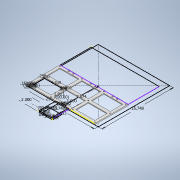
# Autodesk Inventor part: WellPlateFrame - 3L - Part2
Saved by Autodesk Inventor 2020 (Build 240168000, 168)
## iProperties
Created: 2023-02-18
Part Number: WellPlateFrame - 3L - Part2
Material: Generic
Document SubType Name: Modeling
Designer: Beaucage
Density: 1 g/cm^3
Appearance: Default
Author: Beaucage
Autodesk Inventor part; units mm, degrees
ref_plane "YZ Plane" through (0, 0, 0) normal (1, 0, 0) x (0, 1, 0)
ref_plane "XZ Plane" through (0, 0, 0) normal (0, 1, 0) x (-1, 0, 0)
ref_plane "XY Plane" through (0, 0, 0) normal (0, 0, 1) x (1, 0, 0)
sketch "Sketch1" plane through (0, 0, 0) normal (0, 1, 0) x (-1, 0, 0)
  line L0 (0, 0) -> (76.2, 0)
  line L1 (76.2, 0) -> (76.2, -50.8)
  line L2 (76.2, -50.8) -> (0, -50.8)
  line L3 (0, -50.8) -> (0, 0)
  line L4 (38.1, 0) -> (38.1, -6.35)
  line L5 (38.1, -6.35) -> (12.7, -6.35)
  line L6 (38.1, -6.35) -> (63.5, -6.35)
  line L7 (38.1, -6.35) -> (63.5, -6.35) construction
  line L8 (63.5, -6.35) -> (63.5, -19.05)
  line L9 (12.7, -6.35) -> (12.7, -19.05)
  line L10 (63.5, -19.05) -> (63.5, -25.4)
  line L11 (12.7, -19.05) -> (12.7, -25.4)
  line L12 (63.5, -19.05) -> (63.5, -94.05)
  line L13 (63.5, -19.05) -> (138.5, -19.05) construction
  line L14 (12.7, -19.05) -> (12.7, -94.05)
  line L15 (63.5, -94.05) -> (38.1, -94.05)
  line L16 (38.1, -94.05) -> (38.1, -294.05)
  line L17 (38.1, -94.05) -> (238.1, -94.05) construction
  line L18 (238.1, -494.05) -> (-161.9, -494.05)
  line L19 (-161.9, -494.05) -> (-161.9, -94.05)
  line L20 (-161.9, -94.05) -> (238.1, -94.05)
  line L21 (238.1, -94.05) -> (238.1, -494.05)
  line L22 (238.1, -494.05) -> (-161.9, -94.05) construction
  line L23 (-161.9, -494.05) -> (238.1, -94.05) construction
  point P0 (63.5, -50.8)
  point P1 (12.7, -50.8)
  dimension "d0" = 76.2
  dimension "d1" = 50.8
  dimension "d2" = 6.35
  dimension "d3" = 25.4
  dimension "d4" = 25.4
  dimension "d5" = 0
  dimension "d6" = 12.7
  dimension "d7" = 12.7
  dimension "d8" = 6.35
  dimension "d9" = 6.35
  dimension "d10" = 75
  dimension "d11" = 90
  dimension "d12" = 75
  dimension "d13" = 25.4
  dimension "d14" = 200
  dimension "d15" = 90
  dimension "d16" = 400
  dimension "d17" = 400
  constraints: 48 end point, 7 horizontal, 6 vertical, 4 parallel, 4 perpendicular, 3 equal length, 3 midpoint, 1 point on line
  measures "d0" distance of L1.end L2.end
  measures "d1" distance of L0.end L1.end
  measures "d2" distance of L4.start L4.end
  measures "d3" distance of L4.end L5.end
  measures "d4" distance of L4.end L6.end
  measures "d5" distance between parallel lines of L6 L7
  measures "d6" distance of L6.end L8.end
  measures "d7" distance of L5.end L9.end
  measures "d8" distance of L8.end L10.end
  measures "d9" distance of L9.end L11.end
  measures "d10" distance of L8.end L12.end
  measures "d11" angle of L12 L13
  measures "d12" distance of L9.end L14.end
  measures "d13" distance of L12.end L15.end
  measures "d14" distance of L15.end L16.end
  measures "d15" angle of L16 L17
  measures "d16" distance of L19.end L20.end
  measures "d17" distance of L18.end L19.end
extrude "Extrusion1" add sketch "Sketch1" along normal blind 6.35
hole "Hole1" at (-12.7, 0, -6.35) at (-12.7, 0, -19.05) at (-63.5, 0, -6.35) at (-63.5, 0, -19.05) direction (0, 1, 0) diameter 6.604 end through all
sketch "Sketch2" plane through (0, 0, 0) normal (0, -1, 0) x (1, 0, 0)
  line L0 (-238.1, -94.05) -> (-63.5, -94.05) projected
  line L1 (-238.1, -94.05) -> (-238.1, -100.4)
  line L2 (-238.1, -94.05) -> (-231.75, -94.05) construction
  line L3 (-238.1, -100.4) -> (-231.75, -100.4)
  line L4 (-231.75, -100.4) -> (-225.4, -100.4)
  line L5 (-225.4, -100.4) -> (-225.4, -106.75)
  line L6 (-225.4, -106.75) -> (-115.2, -106.75)
  line L7 (-115.2, -106.75) -> (-115.2, -180.75)
  line L8 (-115.2, -180.75) -> (-225.4, -180.75)
  line L9 (-225.4, -180.75) -> (-225.4, -106.75)
  line L10 (-115.2, -106.75) -> (-115.2, -100.4)
  line L11 (-115.2, -100.4) -> (-108.85, -100.4)
  line L12 (-225.4, -180.75) -> (-231.75, -180.75)
  line L13 (-231.75, -180.75) -> (-231.75, -187.1)
  line L14 (-115.2, -180.75) -> (-115.2, -187.1)
  line L15 (-115.2, -187.1) -> (-108.85, -187.1)
  line L16 (-225.4, -106.75) -> (-225.4, -114.75)
  line L17 (-225.4, -106.75) -> (-217.4, -106.75) construction
  line L18 (-225.4, -106.75) -> (-223.4, -106.75)
  line L19 (-223.4, -106.75) -> (-223.4, -108.75)
  line L20 (-223.4, -108.75) -> (-225.4, -108.75)
  line L21 (-225.4, -108.75) -> (-225.4, -106.75)
  line L22 (-115.2, -180.75) -> (-117.2, -180.75)
  line L23 (-117.2, -180.75) -> (-117.2, -178.75)
  line L24 (-117.2, -178.75) -> (-115.2, -178.75)
  line L25 (-115.2, -178.75) -> (-115.2, -180.75)
  line L26 (-223.4, -108.75) -> (-117.2, -108.75)
  line L27 (-117.2, -108.75) -> (-117.2, -178.75)
  line L28 (-117.2, -178.75) -> (-223.4, -178.75)
  line L29 (-223.4, -178.75) -> (-223.4, -108.75)
  point P0 (0, 0)
  dimension "d27" = 6.35
  dimension "d28" = 90
  dimension "d29" = 6.35
  dimension "d30" = 6.35
  dimension "d31" = 6.35
  dimension "d32" = 110.2
  dimension "d33" = 74
  dimension "d34" = 6.35
  dimension "d35" = 6.35
  dimension "d36" = 6.35
  dimension "d37" = 6.35
  dimension "d38" = 6.35
  dimension "d39" = 8
  dimension "d40" = 90
  dimension "d41" = 2
  dimension "d42" = 2
  dimension "d43" = 2
  dimension "d44" = 2
  constraints: 58 end point, 11 perpendicular, 8 horizontal, 8 parallel, 4 vertical
  measures "d27" distance of L0.start L1.end
  measures "d28" angle of L1 L2
  measures "d29" distance of L1.end L3.end
  measures "d30" distance of L3.end L4.end
  measures "d31" distance of L4.end L5.end
  measures "d32" distance of L7.end L8.end
  measures "d33" distance of L6.end L7.end
  measures "d34" distance of L10.end L11.end
  measures "d35" distance of L8.end L12.end
  measures "d36" distance of L12.end L13.end
  measures "d37" distance of L7.end L14.end
  measures "d38" distance of L14.end L15.end
  measures "d39" distance of L5.end L16.end
  measures "d40" angle of L16 L17
  measures "d41" distance of L19.end L20.end
  measures "d42" distance of L18.end L19.end
  measures "d43" distance of L23.end L24.end
  measures "d44" distance of L22.end L23.end
extrude "Extrusion2" cut sketch "Sketch2" against normal through all contours L26 L27 L28 L29
hole "Hole2" at (-231.75, 0, -100.4) at (-231.75, 0, -187.1) at (-108.85, 0, -100.4) at (-108.85, 0, -187.1) direction (0, 1, 0) diameter 5.1562 end through all
extrude "Extrusion3" cut sketch "Sketch2" against normal blind 2 contours L6 L19 L20 L9 | L6 L7 L24 L27 L26 L19 | L20 L29 L28 L23 L8 L9 | L7 L8 L23 L24
pattern_linear "Rectangular Pattern1" count 3 spacing 122.9106 along (1, 0, 0) count 4 spacing 86.9442 along (0, 0, -1) of "Extrusion2", "Hole2", "Extrusion3"
sketch "Sketch3" plane through (0, 0, 0) normal (0, -1, 0) x (1, 0, 0)
  circle A0 centre (136.9712, -447.9326) radius 2.5781 projected
  line L0 (136.9712, -447.9326) -> (143.3212, -447.9326)
  line L1 (143.3212, -447.9326) -> (143.3212, -454.2826)
  line L2 (143.3212, -454.2826) -> (136.9712, -454.2826)
  line L3 (136.9712, -454.2826) -> (136.9712, -447.9326)
  line L4 (-12.7, -94.05) -> (161.9, -94.05) projected
  line L5 (143.3212, -454.2826) -> (161.9, -454.2826)
  line L6 (161.9, -454.2826) -> (161.9, -94.05)
  line L7 (161.9, -94.05) -> (143.3212, -94.05)
  line L8 (143.3212, -94.05) -> (143.3212, -454.2826)
  line L9 (161.9, -454.2826) -> (-238.1, -454.2826)
  line L10 (-238.1, -454.2826) -> (-238.1, -500.3541)
  line L11 (-238.1, -500.3541) -> (161.9, -500.3541)
  line L12 (161.9, -500.3541) -> (161.9, -454.2826)
  point P0 (0, 0)
  dimension "d62" = 6.35
  dimension "d63" = 6.35
  constraints: 24 end point, 6 parallel, 3 horizontal, 3 perpendicular
  measures "d62" distance of L1.end L2.end
  measures "d63" distance of L0.end L1.end
extrude "Extrusion4" cut sketch "Sketch3" against normal through all contours L8 L4 L6 L5 L1 | L2 L5 L12 L11 L10 L9
sketch "Sketch4" plane through (0, 6.35, 0) normal (0, 1, 0) x (1, 0, 0)
  line L0 (-12.7, 94.05) -> (143.3212, 94.05) projected
  line L1 (-76.2, 0) -> (0, 0)
  line L2 (0, 0) -> (0, 94.05)
  line L3 (0, 94.05) -> (-76.2, 94.05)
  line L4 (-76.2, 94.05) -> (-76.2, 0)
  line L5 (-38.1, 94.05) -> (-38.1, 100.4)
  line L6 (-38.1, 100.4) -> (-25.4, 100.4)
  line L7 (-25.4, 100.4) -> (-50.8, 100.4)
  line L8 (-238.1, 454.2826) -> (143.3212, 454.2826)
  line L9 (143.3212, 454.2826) -> (143.3212, 280.6384)
  line L10 (143.3212, 280.6384) -> (-238.1, 280.6384)
  line L11 (-238.1, 280.6384) -> (-238.1, 454.2826)
  dimension "d66" = 6.35
  dimension "d67" = 12.7
  dimension "d68" = 25.4
  constraints: 22 end point, 4 parallel, 3 perpendicular, 2 horizontal, 2 point on line, 1 midpoint, 1 vertical
  measures "d66" distance of L5.start L5.end
  measures "d67" distance of L5.end L6.end
  measures "d68" distance of L6.end L7.end
extrude "Extrusion5" cut sketch "Sketch4" against normal blind 25.4 contours L0 L2 L1 L4 L3
hole "Hole3" at (-50.8, 6.35, -100.4) at (-25.4, 6.35, -100.4) direction (0, -1, 0) diameter 6.7564 end through all clearance for "Socket Head Cap Screw" size "1/4" standard "Ansi Unified Screw Threads"
sketch "Sketch5" plane through (-238.1, 6.35, -94.05) normal (0, 0, 1) x (1, 0, 0)
  line L0 (200, 0) -> (200, -3.175)
  line L1 (174.6, -1.5875) -> (225.4, -1.5875)
  line L2 (225.4, -1.5875) -> (225.4, -4.7625)
  line L3 (225.4, -4.7625) -> (174.6, -4.7625)
  line L4 (174.6, -4.7625) -> (174.6, -1.5875)
  line L5 (174.6, -1.5875) -> (225.4, -4.7625) construction
  line L6 (225.4, -1.5875) -> (174.6, -4.7625) construction
  point P0 (238.1, -6.35)
  dimension "d78" = 3.175
  dimension "d79" = 50.8
  dimension "d80" = 3.175
  constraints: 14 end point, 2 midpoint, 2 parallel, 1 horizontal, 1 perpendicular, 1 vertical
  measures "d78" distance of L0.start L0.end
  measures "d79" distance of L2.end L3.end
  measures "d80" distance of L1.end L2.end
extrude "Extrusion6" cut sketch "Sketch5" against normal blind 3.175
extrude "Extrusion7" cut sketch "Sketch4" against normal blind 31.75 contours L8 L9 L10 L11
sketch "Sketch6" plane through (143.3212, 0, -280.6384) normal (0, 0, -1) x (-1, 0, 0)
  line L0 (120.9, 6.35) -> (14.7, 6.35) projected
  line L1 (243.8106, 6.35) -> (137.6106, 6.35) projected
  line L2 (366.7212, 6.35) -> (260.5212, 6.35) projected
  line L3 (368.7212, 2) -> (258.5212, 2) projected
  line L4 (243.8106, 2) -> (137.6106, 2) projected
  line L5 (137.6106, 6.35) -> (243.8106, 6.35) projected
  line L6 (14.7, 6.35) -> (120.9, 6.35) projected
  line L7 (120.9, 2) -> (14.7, 2) projected
  line L8 (243.8106, 2) -> (137.6106, 2)
  line L9 (137.6106, 2) -> (190.743, 2)
  line L10 (190.743, 0) -> (190.743, 6.35) projected
  line L11 (190.743, 6.35) -> (197.4994, 6.35) projected
  line L12 (190.743, 6.35) -> (190.743, 3.175)
  line L13 (165.343, 1.5875) -> (216.143, 1.5875)
  line L14 (216.143, 1.5875) -> (216.143, 4.7625)
  line L15 (216.143, 4.7625) -> (165.343, 4.7625)
  line L16 (165.343, 4.7625) -> (165.343, 1.5875)
  line L17 (165.343, 1.5875) -> (216.143, 4.7625) construction
  line L18 (216.143, 1.5875) -> (165.343, 4.7625) construction
  line L19 (14.7, 2) -> (14.7, 6.35) projected
  line L20 (14.7, 2) -> (120.9, 2) projected
  line L21 (14.7, 2) -> (120.9, 2)
  line L22 (120.9, 2) -> (67.8, 2)
  line L23 (120.9, 6.35) -> (14.7, 6.35) projected
  line L24 (67.8, 6.35) -> (67.8, 3.175)
  line L25 (42.4, 1.5875) -> (93.2, 1.5875)
  line L26 (93.2, 1.5875) -> (93.2, 4.7625)
  line L27 (93.2, 4.7625) -> (42.4, 4.7625)
  line L28 (42.4, 4.7625) -> (42.4, 1.5875)
  line L29 (42.4, 1.5875) -> (93.2, 4.7625) construction
  line L30 (93.2, 1.5875) -> (42.4, 4.7625) construction
  line L31 (258.5212, 2) -> (368.7212, 2) projected
  line L32 (313.6212, 2) -> (313.6212, 6.35)
  line L33 (313.6212, 6.35) -> (313.6212, 3.175)
  line L34 (288.2212, 1.5875) -> (339.0212, 1.5875)
  line L35 (339.0212, 1.5875) -> (339.0212, 4.7625)
  line L36 (339.0212, 4.7625) -> (288.2212, 4.7625)
  line L37 (288.2212, 4.7625) -> (288.2212, 1.5875)
  line L38 (288.2212, 1.5875) -> (339.0212, 4.7625) construction
  line L39 (339.0212, 1.5875) -> (288.2212, 4.7625) construction
  point P0 (143.3212, 0)
  dimension "d85" = 3.175
  dimension "d86" = 50.8
  dimension "d87" = 3.175
  dimension "d88" = 3.175
  dimension "d89" = 50.8
  dimension "d90" = 3.175
  dimension "d91" = 3.175
  dimension "d92" = 50.8
  dimension "d93" = 3.175
  constraints: 52 end point, 11 midpoint, 7 equal length, 4 horizontal, 3 perpendicular, 3 point on line, 1 vertical
  measures "d85" distance of L10.end L12.end
  measures "d86" distance of L15.end L14.end
  measures "d87" distance of L14.end L13.end
  measures "d88" distance of L24.start L24.end
  measures "d89" distance of L27.end L26.end
  measures "d90" distance of L26.end L25.end
  measures "d91" distance of L32.end L33.end
  measures "d92" distance of L36.end L35.end
  measures "d93" distance of L35.end L34.end
extrude "Extrusion8" add sketch "Sketch6" along normal blind 3.175 contours L27 L26 L7 L28 | L7 L26 L25 L28 | L35 L34 L37 L3 | L3 L32 L36 L35 | L3 L37 L36 L32 | L14 L13 L10 L4 | L4 L10 L15 L14 | L10 L13 L16 L4 | L4 L16 L15 L10
sketch "Sketch7" plane through (0, 6.35, 0) normal (0, 1, 0) x (1, 0, 0)
  line L0 (50.1212, 283.8134) -> (100.9212, 283.8134) projected
  line L1 (75.5212, 283.8134) -> (75.5212, 274.2884)
  line L2 (75.5212, 274.2884) -> (62.8212, 274.2884)
  line L3 (62.8212, 274.2884) -> (88.2212, 274.2884)
  line L4 (-22.0218, 283.8134) -> (-72.8218, 283.8134) projected
  line L5 (-47.4218, 283.8134) -> (-47.4218, 274.2884)
  line L6 (-47.4218, 274.2884) -> (-60.1218, 274.2884)
  line L7 (-60.1218, 274.2884) -> (-34.7218, 274.2884)
  line L8 (-144.9, 283.8134) -> (-195.7, 283.8134) projected
  line L9 (-170.3, 283.8134) -> (-170.3, 274.2884)
  line L10 (-170.3, 274.2884) -> (-183, 274.2884)
  line L11 (-183, 274.2884) -> (-157.6, 274.2884)
  point P0 (0, 0)
  dimension "d96" = 9.525
  dimension "d97" = 12.7
  dimension "d98" = 25.4
  dimension "d99" = 9.525
  dimension "d100" = 12.7
  dimension "d101" = 25.4
  dimension "d102" = 12.7
  dimension "d103" = 25.4
  constraints: 18 end point, 3 midpoint, 3 perpendicular, 3 point on line, 3 vertical
  measures "d96" distance of L1.start L1.end
  measures "d97" distance of L1.end L2.end
  measures "d98" distance of L2.end L3.end
  measures "d99" distance of L5.start L5.end
  measures "d100" distance of L5.end L6.end
  measures "d101" distance of L6.end L7.end
  measures "d102" distance of L9.end L10.end
  measures "d103" distance of L10.end L11.end
hole "Hole4" at (-183, 6.35, -274.2884) at (-157.6, 6.35, -274.2884) at (-60.1218, 6.35, -274.2884) at (-34.7218, 6.35, -274.2884) at (88.2212, 6.35, -274.2884) at (62.8212, 6.35, -274.2884) direction (0, -1, 0) diameter 6.7564 end through all clearance for "Socket Head Cap Screw" size "1/4" standard "Ansi Unified Screw Threads"
body "Solid1"
